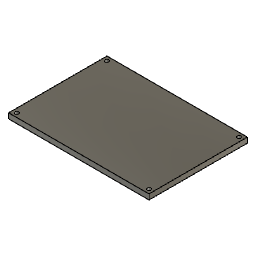
Breadboard Board v1 (Autodesk Fusion 360 design; units mm, degrees)
Autodesk Fusion 360 part; units mm, degrees
sketch "Sketch1" plane through (0, 0, 0) normal (0, 0, 1) x (1, 0, 0)
  line L0 (-60.9615, 37.7743) -> (32.5385, 37.7743)
  line L1 (32.5385, 37.7743) -> (32.5385, -27.7257)
  line L2 (32.5385, -27.7257) -> (-60.9615, -27.7257)
  line L3 (-60.9615, -27.7257) -> (-60.9615, 37.7743)
  circle A0 centre (-58.2115, 35.0243) radius 1.25
  circle A1 centre (29.7885, 35.0243) radius 1.25
  circle A2 centre (-58.2115, -24.9757) radius 1.25
  circle A3 centre (29.7885, -24.9757) radius 1.25
  dimension "d1" = 93.5
  dimension "d2" = 65.5
  dimension "d3" = 2.5
  dimension "d4" = 2.5
  dimension "d5" = 2.5
  dimension "d6" = 2.5
  dimension "d7" = 2.75
  dimension "d8" = 2.75
  dimension "d9" = 2.75
  dimension "d10" = 2.75
  dimension "d11" = 2.75
  dimension "d12" = 2.75
  dimension "d13" = 2.75
  dimension "d14" = 2.75
  constraint horizontal L0
  constraint vertical L1
  constraint horizontal L2
  constraint vertical L3
  measures "d1" distance of L0.start L0.end
  measures "d2" distance of L0.start L2.end
  measures "d3" diameter of A0
  measures "d4" diameter of A1
  measures "d5" diameter of A2
  measures "d6" diameter of A3
  measures "d7" distance of L0 A0.centre
  measures "d8" distance of L3 A0.centre
  measures "d9" distance of L0 A1.centre
  measures "d10" distance of L1 A1.centre
  measures "d11" distance of L1 A3.centre
  measures "d12" distance of L2 A3.centre
  measures "d13" distance of L2 A2.centre
  measures "d14" distance of L3 A2.centre
extrude "Extrude1" add sketch "Sketch1" along normal blind 3.5
